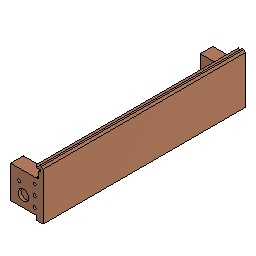
side_right (Autodesk Fusion 360 design; units mm, degrees)
Autodesk Fusion 360 part; units mm, degrees
note: some values were not read from the file. Set by a fixed rule: which sketch regions a step uses.
sketch "Skizze1" plane through (0, 0, 0) normal (0, 1, 0) x (1, 0, 0)
  line L0 (0, -95.7521) -> (0, 79.6341) construction
  line L1 (0, 0) -> (0, -57.828)
  line L2 (-44, 0) -> (25, 0) construction
  line L3 (0, -57.828) -> (-4, -57.828)
  line L4 (-10.2207, -51.6073) -> (4.586, -66.414) construction
  line L5 (-4, -57.828) -> (-6.8284, -54.9996)
  line L6 (-6.8284, -54.9996) -> (-8.243, -56.4141)
  line L7 (-8.243, -56.4141) -> (-8.243, 0)
  line L8 (-8.243, 0) -> (0, 0)
  line L9 (-8.243, -53.585) -> (-5.243, -53.585)
  line L10 (-5.243, -53.585) -> (-3.243, -53.585)
  line L11 (-3.243, -53.585) -> (-3.243, -51.585)
  line L12 (-3.243, -51.585) -> (-5.243, -51.585)
  line L13 (-5.243, -51.585) -> (-5.243, -53.585)
  line L14 (-8.243, -43.585) -> (-12.058, -43.585)
  line L15 (-12.058, -43.585) -> (-8.243, -53.585)
  line L16 (-8.243, -43.585) -> (-5.243, -43.585)
  line L17 (-5.243, -51.585) -> (-5.243, -43.585)
  dimension "d1" = 57.828
  dimension "d2" = 4
  dimension "d3" = 45
  dimension "d4" = 4
  dimension "d5" = 8.243
  dimension "d6" = 4.243
  dimension "d7" = 2
  dimension "d8" = 2
  dimension "d9" = 3
  dimension "d10" = 3.815
  dimension "d11" = 10
  dimension "d17" = 14.243
  dimension "d18" = 43.585
  constraint vertical L0
  constraint coincident L1.start L0
  constraint coincident L1.start L8.end
  constraint coincident L0 L1.end
  constraint horizontal L2
  constraint coincident L1.start L2
  constraint perpendicular L0 L3
  constraint coincident L3.end L4
  constraint coincident L4 L5.end
  constraint perpendicular L5 L6
  constraint vertical L7
  constraint coincident L6.end L7.start
  constraint coincident L2 L7.end
  constraint coincident L7 L9.start
  constraint perpendicular L7 L9
  constraint horizontal L10
  constraint vertical L11
  constraint horizontal L12
  constraint vertical L13
  constraint coincident L7 L14.start
  constraint perpendicular L7 L14
  constraint perpendicular L7 L16
  constraint perpendicular L16 L17
  constraint coincident L16.end L17.end
  measures "d1" distance of L1.end L2
  measures "d2" distance of L0 L3.end
  measures "d3" angle of L0 L4
  measures "d4" distance of L3.end L5.end
  measures "d5" distance of L0 L7
  measures "d6" distance of L3 L9
  measures "d7" distance of L11 L13
  measures "d8" distance of L10 L12
  measures "d9" distance of L7 L9.end
  measures "d10" distance of L7 L14.end
  measures "d11" distance of L9.start L14.start
  measures "d17" distance of L3 L16
  measures "d18" distance of L2 L16.end
extrude "Extrusion1" add sketch "Skizze1" along normal blind 238 contours L1 L3 L5 L6 L7 L8 L9 L10 L11 L12 L16 L17
chamfer "Fase1" distance 2 angle 45 1 edges at (0, 119, 57.828)
ref_plane "Arbeitsebene1" through (-8.243, 0, 0) normal (1, 0, 0) x (0, 1, 0)
sketch "Skizze2" plane through (-8.243, 0, 0) normal (1, 0, 0) x (0, 1, 0)
  line L0 (267.8707, 0) -> (-22.3676, 0) construction
  line L1 (119, 85.1041) -> (119, -43.9964) construction
  line L2 (0, 97.1577) -> (0, -47.4856) construction
  line L3 (274.9535, 43.585) -> (-31.1829, 43.585) construction
  line L4 (115.5, 43.585) -> (122.5, 43.585)
  line L5 (122.5, 43.585) -> (122.5, 50.463)
  line L6 (122.5, 50.463) -> (115.5, 50.463)
  line L7 (115.5, 50.463) -> (115.5, 43.585)
  line L8 (115.5, 43.585) -> (122.5, 50.463) construction
  line L9 (122.5, 43.585) -> (115.5, 50.463) construction
  line L10 (267.9623, 50.463) -> (-13.8401, 50.463) construction
  line L11 (203.5, 43.585) -> (210.5, 43.585)
  line L12 (210.5, 43.585) -> (210.5, 50.463)
  line L13 (210.5, 50.463) -> (203.5, 50.463)
  line L14 (203.5, 50.463) -> (203.5, 43.585)
  line L15 (203.5, 43.585) -> (210.5, 50.463) construction
  line L16 (210.5, 43.585) -> (203.5, 50.463) construction
  line L17 (28.5, 43.585) -> (35.5, 43.585)
  line L18 (35.5, 43.585) -> (35.5, 50.463)
  line L19 (35.5, 50.463) -> (28.5, 50.463)
  line L20 (28.5, 50.463) -> (28.5, 43.585)
  line L21 (28.5, 43.585) -> (35.5, 50.463) construction
  line L22 (35.5, 43.585) -> (28.5, 50.463) construction
  line L23 (220, 68.3899) -> (220, -18.0018) construction
  line L24 (20, 66.908) -> (20, -20) construction
  line L25 (85, 65.5036) -> (85, 11.088) construction
  line L26 (155, 67.0596) -> (155, 11.5194) construction
  line L27 (250.7349, 48.499) -> (-43.738, 48.499) construction
  circle A0 centre (155, 48.499) radius 1.25
  circle A1 centre (85, 48.499) radius 1.25
  circle A2 centre (20, 48.499) radius 1.25
  circle A3 centre (220, 48.499) radius 1.25
  line L28 (21.2702, 46.299) -> (22.5403, 48.499)
  line L29 (22.5403, 48.499) -> (21.2702, 50.699)
  line L30 (21.2702, 50.699) -> (18.7298, 50.699)
  line L31 (18.7298, 50.699) -> (17.4597, 48.499)
  line L32 (17.4597, 48.499) -> (18.7298, 46.299)
  line L33 (18.7298, 46.299) -> (21.2702, 46.299)
  line L34 (86.2702, 46.299) -> (87.5403, 48.499)
  line L35 (87.5403, 48.499) -> (86.2702, 50.699)
  line L36 (86.2702, 50.699) -> (83.7298, 50.699)
  line L37 (83.7298, 50.699) -> (82.4597, 48.499)
  line L38 (82.4597, 48.499) -> (83.7298, 46.299)
  line L39 (83.7298, 46.299) -> (86.2702, 46.299)
  line L40 (156.2702, 46.299) -> (157.5403, 48.499)
  line L41 (157.5403, 48.499) -> (156.2702, 50.699)
  line L42 (156.2702, 50.699) -> (153.7298, 50.699)
  line L43 (153.7298, 50.699) -> (152.4597, 48.499)
  line L44 (152.4597, 48.499) -> (153.7298, 46.299)
  line L45 (153.7298, 46.299) -> (156.2702, 46.299)
  line L46 (221.2702, 46.299) -> (222.5403, 48.499)
  line L47 (222.5403, 48.499) -> (221.2702, 50.699)
  line L48 (221.2702, 50.699) -> (218.7298, 50.699)
  line L49 (218.7298, 50.699) -> (217.4597, 48.499)
  line L50 (217.4597, 48.499) -> (218.7298, 46.299)
  line L51 (218.7298, 46.299) -> (221.2702, 46.299)
  line L52 (238, 80) -> (238, -10) construction
  line L53 (223, 43) -> (223, 20)
  line L54 (223, 20) -> (193, 20)
  line L55 (223, 43) -> (238, 43)
  line L56 (15, 43) -> (0, 43)
  line L57 (15, 43) -> (15, 20)
  line L58 (15, 20) -> (45, 20)
  line L59 (238, 43) -> (238, 5)
  line L60 (238, 5) -> (193, 5)
  line L61 (193, 20) -> (193, 5)
  line L62 (45, 20) -> (45, 5)
  line L63 (0, 5) -> (45, 5)
  line L64 (0, 43) -> (0, 5)
  line L65 (66.5, 43.585) -> (63.5, 43.585) construction
  line L66 (63.5, 43.585) -> (63.5, 48.585)
  line L67 (60.5, 51.585) -> (69.5, 51.585)
  line L68 (66.5, 48.585) -> (66.5, 43.585)
  line L69 (66.5, 43.585) -> (63.5, 43.585) construction
  line L70 (63.5, 43.585) -> (63.5, 33.585)
  line L71 (66.5, 33.585) -> (66.5, 43.585)
  line L72 (65, 56) -> (65, 28) construction
  arc A4 (63.5, 33.585) -> (66.5, 33.585) centre (65, 33.585) ccw
  line L73 (125.8642, 33.585) -> (76, 33.585) construction
  circle A5 centre (58.65, 33.585) radius 4
  circle A6 centre (71.35, 33.585) radius 4
  circle A7 centre (58.65, 33.585) radius 3
  circle A8 centre (71.35, 33.585) radius 3
  line L74 (72.6202, 31.385) -> (73.8903, 33.585)
  line L75 (73.8903, 33.585) -> (72.6202, 35.785)
  line L76 (72.6202, 35.785) -> (70.0798, 35.785)
  line L77 (70.0798, 35.785) -> (68.8097, 33.585)
  line L78 (68.8097, 33.585) -> (70.0798, 31.385)
  line L79 (70.0798, 31.385) -> (72.6202, 31.385)
  line L80 (59.9202, 31.385) -> (61.1903, 33.585)
  line L81 (61.1903, 33.585) -> (59.9202, 35.785)
  line L82 (59.9202, 35.785) -> (57.3798, 35.785)
  line L83 (57.3798, 35.785) -> (56.1097, 33.585)
  line L84 (56.1097, 33.585) -> (57.3798, 31.385)
  line L85 (57.3798, 31.385) -> (59.9202, 31.385)
  circle A9 centre (71.35, 33.585) radius 1.25
  circle A10 centre (58.65, 33.585) radius 1.25
  arc A11 (69.5, 51.585) -> (66.5, 48.585) centre (69.5, 48.585) ccw
  arc A12 (63.5, 48.585) -> (60.5, 51.585) centre (60.5, 48.585) ccw
  line L86 (192, 26.585) -> (129, 26.585) construction
  line L87 (99, 16.585) -> (129, 16.585) construction
  line L88 (129, 16.585) -> (129, 36.585) construction
  line L89 (129, 36.585) -> (99, 36.585) construction
  line L90 (99, 36.585) -> (99, 16.585) construction
  line L91 (129, 36.585) -> (139, 36.585) construction
  line L92 (139, 36.585) -> (139, 16.585) construction
  line L93 (139, 16.585) -> (129, 16.585) construction
  line L94 (129, 16.585) -> (129, 36.585) construction
  circle A13 centre (99, 26.585) radius 1.25
  circle A14 centre (99, 26.585) radius 4
  circle A15 centre (129, 16.585) radius 1.25
  circle A16 centre (129, 16.585) radius 4
  circle A17 centre (129, 36.585) radius 1.25
  circle A18 centre (129, 36.585) radius 4
  line L95 (130.2702, 34.385) -> (131.5403, 36.585)
  line L96 (131.5403, 36.585) -> (130.2702, 38.785)
  line L97 (130.2702, 38.785) -> (127.7298, 38.785)
  line L98 (127.7298, 38.785) -> (126.4597, 36.585)
  line L99 (126.4597, 36.585) -> (127.7298, 34.385)
  line L100 (127.7298, 34.385) -> (130.2702, 34.385)
  line L101 (130.2702, 14.385) -> (131.5403, 16.585)
  line L102 (131.5403, 16.585) -> (130.2702, 18.785)
  line L103 (130.2702, 18.785) -> (127.7298, 18.785)
  line L104 (127.7298, 18.785) -> (126.4597, 16.585)
  line L105 (126.4597, 16.585) -> (127.7298, 14.385)
  line L106 (127.7298, 14.385) -> (130.2702, 14.385)
  line L107 (100.2702, 24.385) -> (101.5403, 26.585)
  line L108 (101.5403, 26.585) -> (100.2702, 28.785)
  line L109 (100.2702, 28.785) -> (97.7298, 28.785)
  line L110 (97.7298, 28.785) -> (96.4597, 26.585)
  line L111 (96.4597, 26.585) -> (97.7298, 24.385)
  line L112 (97.7298, 24.385) -> (100.2702, 24.385)
  line L113 (99, 36.585) -> (129, 16.585) construction
  line L114 (129, 36.585) -> (99, 16.585) construction
  point P0 (119, 47.024)
  point P1 (207, 47.024)
  point P2 (32, 47.024)
  point P3 (20, 48.499)
  point P4 (85, 48.499)
  point P5 (155, 48.499)
  point P6 (220, 48.499)
  point P7 (68.35, 33.585)
  point P8 (61.65, 33.585)
  point P9 (71.35, 33.585)
  point P10 (58.65, 33.585)
  point P11 (155, 26.585)
  point P12 (129, 36.585)
  point P13 (129, 16.585)
  point P14 (99, 26.585)
  point P15 (114, 26.585)
  dimension "d16" = 119
  dimension "d19" = 43.585
  dimension "d20" = 7
  dimension "d22" = 6.878
  dimension "d23" = 7
  dimension "d24" = 7
  dimension "d25" = 88
  dimension "d26" = 87
  dimension "d27" = 101
  dimension "d28" = 99
  dimension "d30" = 34
  dimension "d32" = 36
  dimension "d33" = 4.914
  dimension "d34" = 2.5
  dimension "d35" = 2.5
  dimension "d36" = 2.5
  dimension "d37" = 2.5
  dimension "d38" = 4.4
  dimension "d39" = 4.4
  dimension "d40" = 4.4
  dimension "d41" = 4.4
  dimension "d42" = 119
  dimension "d60" = 15
  dimension "d61" = 38
  dimension "d62" = 5
  dimension "d63" = 15
  dimension "d64" = 45
  dimension "d154" = 8
  dimension "d155" = 3
  dimension "d157" = 1.5
  dimension "d159" = 1.5
  dimension "d162" = 6.35
  dimension "d163" = 8
  dimension "d164" = 10
  dimension "d165" = 6.35
  dimension "d166" = 8
  dimension "d167" = 6
  dimension "d168" = 6
  dimension "d169" = 4.4
  dimension "d170" = 4.4
  dimension "d171" = 2.5
  dimension "d172" = 2.5
  dimension "d177" = 3
  dimension "d178" = 3
  dimension "d189" = 20
  dimension "d190" = 30
  dimension "d191" = 10
  dimension "d192" = 17
  dimension "d193" = 8
  dimension "d194" = 8
  dimension "d195" = 8
  dimension "d196" = 2.5
  dimension "d197" = 2.5
  dimension "d198" = 2.5
  dimension "d199" = 4.4
  dimension "d200" = 4.4
  dimension "d201" = 4.4
  dimension "d204" = 20
  dimension "d205" = 5
  constraint horizontal L0
  constraint coincident origin L0
  constraint perpendicular L0 L1
  constraint perpendicular L0 L2
  constraint coincident origin L2
  constraint perpendicular L1 L3
  constraint horizontal L4
  constraint perpendicular L4 L5
  constraint parallel L4 L6
  constraint parallel L5 L7
  constraint coincident L8 P0
  constraint coincident L9 P0
  constraint coincident L1 P0
  constraint coincident L3 L4.start
  constraint perpendicular L2 L10
  constraint coincident L6.end L10
  constraint horizontal L11
  constraint perpendicular L11 L12
  constraint parallel L11 L13
  constraint parallel L12 L14
  constraint coincident L15 P1
  constraint coincident L16 P1
  constraint horizontal L17
  constraint perpendicular L17 L18
  constraint parallel L17 L19
  constraint parallel L18 L20
  constraint coincident L21 P2
  constraint coincident L22 P2
  constraint coincident L3 L17.start
  constraint coincident L10 L18.end
  constraint coincident L3 L11.start
  constraint coincident L10 L13.end
  constraint perpendicular L3 L23
  constraint perpendicular L10 L24
  constraint perpendicular L10 L25
  constraint perpendicular L3 L26
  constraint perpendicular L2 L27
  constraint coincident L27 P5
  constraint coincident L26 P5
  constraint coincident L27 P4
  constraint coincident L25 P4
  constraint coincident L24 P3
  constraint coincident L27 P3
  constraint coincident L27 P6
  constraint coincident L23 P6
  constraint coincident P3 A2.centre
  constraint coincident P4 A1.centre
  constraint coincident P5 A0.centre
  constraint coincident P6 A3.centre
  constraint horizontal L51
  constraint horizontal L45
  constraint horizontal L39
  constraint horizontal L33
  constraint perpendicular L27 L52
  constraint coincident L52 L55.end
  constraint perpendicular L0 L53
  constraint perpendicular L53 L54
  constraint symmetric L1 L55.end L56.end
  constraint symmetric L1 L53.start L56.start
  constraint symmetric L1 L53.end L57.end
  constraint symmetric L1 L54.end L58.end
  constraint coincident L52 L59.end
  constraint perpendicular L55 L59
  constraint perpendicular L59 L60
  constraint perpendicular L60 L61
  constraint coincident L60.end L61.end
  constraint symmetric L1 L59.end L63.start
  constraint symmetric L1 L60.end L62.end
  constraint horizontal L65
  constraint vertical L66
  constraint horizontal L67
  constraint vertical L68
  constraint coincident L3 L65.start
  constraint horizontal L69
  constraint vertical L70
  constraint vertical L71
  constraint coincident L66 L65.end
  constraint perpendicular L25 L73
  constraint coincident A4.centre L73
  constraint coincident L73 P10
  constraint coincident L71.start L73
  constraint coincident L73 P9
  constraint concentric A5 A7
  constraint concentric A6 A8
  constraint coincident L73 P7
  constraint coincident A8 P7
  constraint coincident L73 P8
  constraint coincident A7 P8
  constraint coincident P9 A6.centre
  constraint coincident P10 A5.centre
  constraint horizontal L85
  constraint horizontal L79
  constraint concentric A8 A9
  constraint concentric A5 A10
  constraint tangent L67 A12
  constraint tangent L66 A12
  constraint tangent L68 A11
  constraint tangent L67 A11
  constraint perpendicular L26 L86
  constraint horizontal L87
  constraint perpendicular L87 L88
  constraint parallel L87 L89
  constraint parallel L88 L90
  constraint coincident L86 P11
  constraint horizontal L91
  constraint vertical L92
  constraint horizontal L93
  constraint vertical L94
  constraint coincident L87 P13
  constraint coincident L26 P11
  constraint midpoint L90 P14
  constraint concentric A13 A14
  constraint coincident P13 L87.end
  constraint concentric A15 A16
  constraint coincident P12 L88.end
  constraint concentric A17 A18
  constraint coincident P14 A13.centre
  constraint horizontal L112
  constraint horizontal L100
  constraint horizontal L106
  constraint midpoint L114 P15
  constraint coincident L86 P15
  measures "d16" distance of L1 L2
  measures "d19" distance of L0 L3
  measures "d20" distance of L5 L7
  measures "d22" distance of L3 L10
  measures "d23" distance of L18 L20
  measures "d24" distance of L12 L14
  measures "d25" distance of L1 P1
  measures "d26" distance of L1 P2
  measures "d27" distance of L1 L23
  measures "d28" distance of L1 L24
  measures "d30" distance of L1 L25
  measures "d32" distance of L1 L26
  measures "d33" distance of L3 L27
  measures "d34" diameter of A3
  measures "d35" diameter of A0
  measures "d36" diameter of A1
  measures "d37" diameter of A2
  measures "d38" distance of L30 L33
  measures "d39" distance of L36 L39
  measures "d40" distance of L42 L45
  measures "d41" distance of L48 L51
  measures "d42" distance of L1 L52
  measures "d60" distance of L54 L60
  measures "d61" distance of L55 L60
  measures "d62" distance of L0 L60
  measures "d63" distance of L53 L59
  measures "d64" distance of L52 L61
  measures "d154" distance of L65 L67
  measures "d155" distance of L66 L68
  measures "d157" distance of L71 L72
  measures "d159" radius of A4
  measures "d162" distance of A4.centre P10
  measures "d163" diameter of A5
  measures "d164" distance of L3 L73
  measures "d165" distance of L72 P9
  measures "d166" diameter of A6
  measures "d167" diameter of A7
  measures "d168" diameter of A8
  measures "d169" distance of L76 L79
  measures "d170" distance of L82 L85
  measures "d171" diameter of A10
  measures "d172" diameter of A9
  measures "d177" radius of A12
  measures "d178" radius of A11
  measures "d189" distance of L87 L89
  measures "d190" distance of L88 L90
  measures "d191" distance of L88 L92
  measures "d192" distance of L3 L86
  measures "d193" diameter of A14
  measures "d194" diameter of A16
  measures "d195" diameter of A18
  measures "d196" diameter of A17
  measures "d197" diameter of A15
  measures "d198" diameter of A13
  measures "d199" distance of L109 L112
  measures "d200" distance of L97 L100
  measures "d201" distance of L103 L106
  measures "d204" distance of L25 L72
  measures "d205" distance of L1 P15
extrude "Extrusion2" cut sketch "Skizze2" along normal blind 5 contours L4 L5 L6 L7 | L11 L12 L13 L14 | L17 L18 L19 L20
move_face "Flächen versetzen1" offset -0.2 13 faces at (-7.243, 149.5, 43.585) (-3.243, 33.1667, 45.8777) (-3.243, 117.8333, 48.1703) (-3.243, 208.1667, 48.1703) (-4.5763, 28.5, 48.1703) (-4.5763, 115.5, 48.1703) (-4.5763, 203.5, 48.1703) (-3.9097, 35.5, 48.1703) (-3.9097, 122.5, 48.1703) (-4.5763, 210.5, 48.1703) (-4.5763, 208.1667, 50.463) (-4.5763, 120.1667, 50.463) (-4.5763, 33.1667, 50.463)
extrude "Extrusion3" cut sketch "Skizze2" along normal blind 7 contours A0 | A1 | A2 | A3
extrude "Extrusion4" cut sketch "Skizze2" along normal blind 7 contours L28 L29 L30 L31 L32 L33 | L34 L35 L36 L37 L38 L39 | L40 L41 L42 L43 L44 L45 | L46 L47 L48 L49 L50 L51
extrude "Extrusion5" add sketch "Skizze2" along normal blind 5.2 contours L28 L29 L30 L31 L32 L33 | L34 L35 L36 L37 L38 L39 | L40 L41 L42 L43 L44 L45 | L46 L47 L48 L49 L50 L51
extrude "Extrusion6" cut sketch "Skizze2" along normal blind 3 contours L28 L29 L30 L31 L32 L33 | L34 L35 L36 L37 L38 L39 | L40 L41 L42 L43 L44 L45 | L46 L47 L48 L49 L50 L51
extrude "Extrusion7" add sketch "Skizze2" against normal blind 30 contours L53 L54 L55 L59 L60 L61 | L56 L57 L58 L62 L63 L64
sketch "Skizze3" plane through (0, 0, 0) normal (0, 1, 0) x (1, 0, 0)
  line L0 (0, -92.2199) -> (0, 12.1785) construction
  line L1 (-68.4756, 0) -> (32.4309, 0) construction
  line L2 (-10, -63.9149) -> (-10, 13.2124) construction
  line L3 (-23, -32.8986) -> (-23, 10) construction
  line L4 (-28.243, -73.6203) -> (-28.243, -17.2743) construction
  circle A0 centre (-10, -12) radius 1.75
  circle A1 centre (-10, -24) radius 1.75
  circle A2 centre (-10, -36) radius 1.75
  line L5 (-11.6743, -33.1) -> (-13.3486, -36)
  line L6 (-13.3486, -36) -> (-11.6743, -38.9)
  line L7 (-11.6743, -38.9) -> (-8.3257, -38.9)
  line L8 (-8.3257, -38.9) -> (-6.6514, -36)
  line L9 (-6.6514, -36) -> (-8.3257, -33.1)
  line L10 (-8.3257, -33.1) -> (-11.6743, -33.1)
  line L11 (-11.6743, -21.1) -> (-13.3486, -24)
  line L12 (-13.3486, -24) -> (-11.6743, -26.9)
  line L13 (-11.6743, -26.9) -> (-8.3257, -26.9)
  line L14 (-8.3257, -26.9) -> (-6.6514, -24)
  line L15 (-6.6514, -24) -> (-8.3257, -21.1)
  line L16 (-8.3257, -21.1) -> (-11.6743, -21.1)
  line L17 (-11.6743, -9.1) -> (-13.3486, -12)
  line L18 (-13.3486, -12) -> (-11.6743, -14.9)
  line L19 (-11.6743, -14.9) -> (-8.3257, -14.9)
  line L20 (-8.3257, -14.9) -> (-6.6514, -12)
  line L21 (-6.6514, -12) -> (-8.3257, -9.1)
  line L22 (-8.3257, -9.1) -> (-11.6743, -9.1)
  circle A3 centre (-23, -18) radius 6
  circle A4 centre (-28.243, -30) radius 1.75
  line L23 (-29.9173, -27.1) -> (-31.5916, -30)
  line L24 (-31.5916, -30) -> (-29.9173, -32.9)
  line L25 (-29.9173, -32.9) -> (-26.5687, -32.9)
  line L26 (-26.5687, -32.9) -> (-24.8944, -30)
  line L27 (-24.8944, -30) -> (-26.5687, -27.1)
  line L28 (-26.5687, -27.1) -> (-29.9173, -27.1)
  line L29 (-11.6743, -38.9) -> (-13.3486, -38.9)
  line L30 (-13.3486, -38.9) -> (-13.3486, -33.1)
  line L31 (-13.3486, -33.1) -> (-11.6743, -33.1)
  line L32 (-11.6743, -26.9) -> (-13.3486, -26.9)
  line L33 (-13.3486, -26.9) -> (-13.3486, -21.1)
  line L34 (-13.3486, -21.1) -> (-11.6743, -21.1)
  line L35 (-11.6743, -14.9) -> (-13.3486, -14.9)
  line L36 (-13.3486, -14.9) -> (-13.3486, -9.1)
  line L37 (-13.3486, -9.1) -> (-11.6743, -9.1)
  line L38 (-29.9173, -32.9) -> (-31.5916, -32.9)
  line L39 (-31.5916, -32.9) -> (-31.5916, -27.1)
  line L40 (-31.5916, -27.1) -> (-29.9173, -27.1)
  point P0 (-10, -36)
  point P1 (-10, -24)
  point P2 (-10, -12)
  point P3 (-23, -18)
  point P4 (-28.243, -30)
  dimension "d65" = 10
  dimension "d66" = 13
  dimension "d67" = 28.243
  dimension "d68" = 12
  dimension "d69" = 12
  dimension "d70" = 12
  dimension "d71" = 3.5
  dimension "d72" = 3.5
  dimension "d73" = 3.5
  dimension "d74" = 5.8
  dimension "d75" = 5.8
  dimension "d76" = 5.8
  dimension "d78" = 12
  dimension "d79" = 18
  dimension "d81" = 3.5
  dimension "d82" = 30
  dimension "d83" = 5.8
  constraint vertical L0
  constraint horizontal L1
  constraint coincident origin L0
  constraint coincident origin L1
  constraint perpendicular L1 L2
  constraint perpendicular L1 L3
  constraint vertical L4
  constraint coincident L2 P2
  constraint coincident L2 P1
  constraint coincident L2 P0
  constraint coincident P0 A2.centre
  constraint coincident P1 A1.centre
  constraint coincident P2 A0.centre
  constraint horizontal L10
  constraint horizontal L16
  constraint horizontal L22
  constraint coincident P3 A3.centre
  constraint coincident L4 P4
  constraint coincident P4 A4.centre
  constraint horizontal L28
  constraint horizontal L29
  constraint vertical L30
  constraint horizontal L31
  constraint horizontal L32
  constraint vertical L33
  constraint horizontal L34
  constraint horizontal L35
  constraint vertical L36
  constraint horizontal L37
  constraint horizontal L38
  constraint vertical L39
  constraint horizontal L40
  constraint coincident L28 L23.start
  constraint coincident L10 L5.start
  constraint coincident L16 L11.start
  constraint coincident L22 L17.start
  constraint coincident L17.end L36
  constraint coincident L11.end L33
  constraint coincident L5.end L30
  constraint coincident L23.end L39
  measures "d65" distance of L0 L2
  measures "d66" distance of L2 L3
  measures "d67" distance of L0 L4
  measures "d68" distance of L1 P2
  measures "d69" distance of P2 P1
  measures "d70" distance of P1 P0
  measures "d71" diameter of A2
  measures "d72" diameter of A1
  measures "d73" diameter of A0
  measures "d74" distance of L19 L22
  measures "d75" distance of L13 L16
  measures "d76" distance of L7 L10
  measures "d78" diameter of A3
  measures "d79" distance of L1 P3
  measures "d81" diameter of A4
  measures "d82" distance of L1 P4
  measures "d83" distance of L25 L28
ref_plane "Arbeitsebene2" through (0, 238, 0) normal (0, 1, 0) x (0, 0, 1)
sketch "Skizze4" plane through (0, 238, 0) normal (0, 1, 0) x (1, 0, 0)
  line L0 (0, -55.469) -> (0, 11.8199) construction
  line L1 (5.4144, 0) -> (-61.5509, 0) construction
  line L2 (-10, -43.3376) -> (-10, 10) construction
  circle A0 centre (-10, -12) radius 1.75
  circle A1 centre (-10, -24) radius 1.75
  circle A2 centre (-10, -36) radius 1.75
  line L3 (-28.243, -50) -> (-28.243, 7) construction
  line L4 (-23, -24.4157) -> (-23, -9.4157) construction
  circle A3 centre (-23, -18) radius 6
  circle A4 centre (-28.243, -30) radius 1.75
  line L5 (-11.6743, -33.1) -> (-13.3486, -36)
  line L6 (-13.3486, -36) -> (-11.6743, -38.9)
  line L7 (-11.6743, -38.9) -> (-8.3257, -38.9)
  line L8 (-8.3257, -38.9) -> (-6.6514, -36)
  line L9 (-6.6514, -36) -> (-8.3257, -33.1)
  line L10 (-8.3257, -33.1) -> (-11.6743, -33.1)
  line L11 (-11.6743, -21.1) -> (-13.3486, -24)
  line L12 (-13.3486, -24) -> (-11.6743, -26.9)
  line L13 (-11.6743, -26.9) -> (-8.3257, -26.9)
  line L14 (-8.3257, -26.9) -> (-6.6514, -24)
  line L15 (-6.6514, -24) -> (-8.3257, -21.1)
  line L16 (-8.3257, -21.1) -> (-11.6743, -21.1)
  line L17 (-11.6743, -9.1) -> (-13.3486, -12)
  line L18 (-13.3486, -12) -> (-11.6743, -14.9)
  line L19 (-11.6743, -14.9) -> (-8.3257, -14.9)
  line L20 (-8.3257, -14.9) -> (-6.6514, -12)
  line L21 (-6.6514, -12) -> (-8.3257, -9.1)
  line L22 (-8.3257, -9.1) -> (-11.6743, -9.1)
  line L23 (-29.9173, -27.1) -> (-31.5916, -30)
  line L24 (-31.5916, -30) -> (-29.9173, -32.9)
  line L25 (-29.9173, -32.9) -> (-26.5687, -32.9)
  line L26 (-26.5687, -32.9) -> (-24.8944, -30)
  line L27 (-24.8944, -30) -> (-26.5687, -27.1)
  line L28 (-26.5687, -27.1) -> (-29.9173, -27.1)
  line L29 (-11.6743, -38.9) -> (-13.3486, -38.9)
  line L30 (-13.3486, -38.9) -> (-13.3486, -33.1)
  line L31 (-13.3486, -33.1) -> (-11.6743, -33.1)
  line L32 (-11.6743, -33.1) -> (-11.6743, -38.9)
  line L33 (-11.6743, -26.9) -> (-13.3486, -26.9)
  line L34 (-13.3486, -26.9) -> (-13.3486, -21.1)
  line L35 (-13.3486, -21.1) -> (-11.6743, -21.1)
  line L36 (-11.6743, -21.1) -> (-11.6743, -26.9)
  line L37 (-11.6743, -14.9) -> (-13.3486, -14.9)
  line L38 (-13.3486, -14.9) -> (-13.3486, -9.1)
  line L39 (-13.3486, -9.1) -> (-11.6743, -9.1)
  line L40 (-11.6743, -9.1) -> (-11.6743, -14.9)
  line L41 (-29.9173, -32.9) -> (-31.5916, -32.9)
  line L42 (-31.5916, -32.9) -> (-31.5916, -27.1)
  line L43 (-31.5916, -27.1) -> (-29.9173, -27.1)
  line L44 (-29.9173, -27.1) -> (-29.9173, -32.9)
  point P0 (-10, -36)
  point P1 (-10, -24)
  point P2 (-10, -12)
  point P3 (-28.243, -30)
  dimension "d94" = 10
  dimension "d95" = 12
  dimension "d96" = 12
  dimension "d97" = 12
  dimension "d98" = 3.5
  dimension "d99" = 3.5
  dimension "d100" = 3.5
  dimension "d101" = 28.243
  dimension "d102" = 13
  dimension "d103" = 12
  dimension "d104" = 18
  dimension "d105" = 3.5
  dimension "d106" = 30
  dimension "d107" = 5.8
  dimension "d108" = 5.8
  dimension "d109" = 5.8
  dimension "d110" = 5.8
  constraint vertical L0
  constraint coincident origin L0
  constraint horizontal L1
  constraint coincident origin L1
  constraint perpendicular L1 L2
  constraint coincident L2 P2
  constraint coincident L2 P1
  constraint coincident L2 P0
  constraint perpendicular L1 L3
  constraint vertical L4
  constraint coincident L4 A3.centre
  constraint coincident L3 P3
  constraint coincident P0 A2.centre
  constraint coincident P1 A1.centre
  constraint coincident P2 A0.centre
  constraint coincident P3 A4.centre
  constraint horizontal L10
  constraint horizontal L16
  constraint horizontal L22
  constraint horizontal L28
  constraint horizontal L29
  constraint vertical L30
  constraint horizontal L31
  constraint vertical L32
  constraint horizontal L33
  constraint vertical L34
  constraint horizontal L35
  constraint vertical L36
  constraint horizontal L37
  constraint vertical L38
  constraint horizontal L39
  constraint vertical L40
  constraint horizontal L41
  constraint vertical L42
  constraint horizontal L43
  constraint vertical L44
  constraint coincident L28 L23.start
  constraint coincident L23.end L42
  constraint coincident L5.end L30
  constraint coincident L10 L5.start
  constraint coincident L16 L11.start
  constraint coincident L11.end L34
  constraint coincident L17.end L38
  constraint coincident L22 L17.start
  measures "d94" distance of L0 L2
  measures "d95" distance of L1 P2
  measures "d96" distance of P2 P1
  measures "d97" distance of P1 P0
  measures "d98" diameter of A0
  measures "d99" diameter of A1
  measures "d100" diameter of A2
  measures "d101" distance of L0 L3
  measures "d102" distance of L2 L4
  measures "d103" diameter of A3
  measures "d104" distance of L1 A3.centre
  measures "d105" diameter of A4
  measures "d106" distance of L1 P3
  measures "d107" distance of L25 L28
  measures "d108" distance of L19 L22
  measures "d109" distance of L13 L16
  measures "d110" distance of L7 L10
extrude "Extrusion8" cut sketch "Skizze3" along normal blind 3 contours A3
extrude "Extrusion12" cut sketch "Skizze4" against normal blind 3 contours A3
move_face "Flächen versetzen2" offset -0.2 2 faces at (-21.235, 3, 16.6397) (-17.0075, 2, 18.2991)
move_face "Flächen versetzen3" offset -0.2 2 faces at (-21.235, 235, 16.6397) (-17.0075, 236, 18.2991)
extrude "Extrusion9" cut sketch "Skizze3" along normal blind 17 contours A0 | A1 | A2 | A4
extrude "Extrusion13" cut sketch "Skizze4" against normal blind 17 contours A0 L40 | A0 L40 | A1 L36 | A1 L36 | A2 L32 | A2 L32 | A4 L44 | A4 L44
extrude "Extrusion10" cut sketch "Skizze3" along normal blind 6 contours L5 L6 L7 L8 L9 L10 | L5 L30 L31 | L6 L29 L30 | L11 L12 L13 L14 L15 L16 | L11 L33 L34 | L12 L32 L33 | L17 L18 L19 L20 L21 L22 | L17 L36 L37 | L18 L35 L36 | L23 L24 L25 L26 L27 L28 | L23 L39 L40 | L24 L38 L39
extrude "Extrusion14" cut sketch "Skizze4" against normal blind 6 contours A0 L19 L20 L21 L22 L40 | A0 L17 L18 L40 | L17 L38 L39 | L18 L37 L38 | A1 L13 L14 L15 L16 L36 | A1 L11 L12 L36 | L11 L34 L35 | L12 L33 L34 | A2 L7 L8 L9 L10 L32 | A2 L5 L6 L32 | L5 L30 L31 | L6 L29 L30 | A4 L25 L26 L27 L28 L44 | A4 L23 L24 L44 | L23 L42 L43 | L24 L41 L42
extrude "Extrusion11" add sketch "Skizze3" along normal blind 3.2 contours L5 L6 L7 L8 L9 L10 | L5 L30 L31 | L6 L29 L30 | L11 L12 L13 L14 L15 L16 | L11 L33 L34 | L12 L32 L33 | L17 L18 L19 L20 L21 L22 | L17 L36 L37 | L18 L35 L36 | L23 L24 L25 L26 L27 L28 | L23 L39 L40 | L24 L38 L39
extrude "Extrusion15" add sketch "Skizze4" against normal blind 3.2 contours A0 L19 L20 L21 L22 L40 | A0 L17 L18 L40 | L17 L38 L39 | L18 L37 L38 | A1 L13 L14 L15 L16 L36 | A1 L11 L12 L36 | L11 L34 L35 | L12 L33 L34 | A2 L7 L8 L9 L10 L32 | A2 L5 L6 L32 | L5 L30 L31 | L6 L29 L30 | A4 L25 L26 L27 L28 L44 | A4 L23 L24 L44 | L23 L42 L43 | L24 L41 L42
ref_plane "Arbeitsebene3" through (0, 0, 5) normal (0, 0, 1) x (1, 0, 0)
sketch "Skizze5" plane through (0, 0, 5) normal (0, 0, 1) x (1, 0, 0)
  line L0 (0, 304.2295) -> (0, -44.6132) construction
  line L1 (40.8968, 0) -> (-125, 0) construction
  line L2 (-16.743, 290) -> (-16.743, -30) construction
  line L3 (-30.743, 288.1348) -> (-30.743, -30) construction
  line L4 (17.6636, 10) -> (-56.9116, 10) construction
  line L5 (15.9426, 35) -> (-60, 35) construction
  line L6 (28.5025, 203) -> (-55.3761, 203) construction
  line L7 (20, 228) -> (-65.678, 228) construction
  line L8 (-12.2276, 194.9367) -> (-36.234, 237.8054) construction
  line L9 (-7.0433, 245.3209) -> (-37.9735, 190.0885) construction
  line L10 (-12.4101, 42.7373) -> (-35.0759, 2.2627) construction
  line L11 (-13.8411, 4.818) -> (-37.2196, 46.5654) construction
  circle A0 centre (-23.743, 22.5) radius 4
  circle A1 centre (-23.743, 215.5) radius 4
  circle A2 centre (-30.743, 10) radius 1.75
  circle A3 centre (-30.743, 35) radius 1.75
  circle A4 centre (-16.743, 35) radius 1.75
  circle A5 centre (-16.743, 10) radius 1.75
  circle A6 centre (-30.743, 228) radius 1.75
  circle A7 centre (-16.743, 228) radius 1.75
  circle A8 centre (-16.743, 203) radius 1.75
  circle A9 centre (-30.743, 203) radius 1.75
  line L12 (-29.0687, 225.1) -> (-27.3944, 228)
  line L13 (-27.3944, 228) -> (-29.0687, 230.9)
  line L14 (-29.0687, 230.9) -> (-32.4173, 230.9)
  line L15 (-32.4173, 230.9) -> (-34.0916, 228)
  line L16 (-34.0916, 228) -> (-32.4173, 225.1)
  line L17 (-32.4173, 225.1) -> (-29.0687, 225.1)
  line L18 (-15.0687, 225.1) -> (-13.3944, 228)
  line L19 (-13.3944, 228) -> (-15.0687, 230.9)
  line L20 (-15.0687, 230.9) -> (-18.4173, 230.9)
  line L21 (-18.4173, 230.9) -> (-20.0916, 228)
  line L22 (-20.0916, 228) -> (-18.4173, 225.1)
  line L23 (-18.4173, 225.1) -> (-15.0687, 225.1)
  line L24 (-15.0687, 200.1) -> (-13.3944, 203)
  line L25 (-13.3944, 203) -> (-15.0687, 205.9)
  line L26 (-15.0687, 205.9) -> (-18.4173, 205.9)
  line L27 (-18.4173, 205.9) -> (-20.0916, 203)
  line L28 (-20.0916, 203) -> (-18.4173, 200.1)
  line L29 (-18.4173, 200.1) -> (-15.0687, 200.1)
  line L30 (-29.0687, 200.1) -> (-27.3944, 203)
  line L31 (-27.3944, 203) -> (-29.0687, 205.9)
  line L32 (-29.0687, 205.9) -> (-32.4173, 205.9)
  line L33 (-32.4173, 205.9) -> (-34.0916, 203)
  line L34 (-34.0916, 203) -> (-32.4173, 200.1)
  line L35 (-32.4173, 200.1) -> (-29.0687, 200.1)
  line L36 (-29.0687, 32.1) -> (-27.3944, 35)
  line L37 (-27.3944, 35) -> (-29.0687, 37.9)
  line L38 (-29.0687, 37.9) -> (-32.4173, 37.9)
  line L39 (-32.4173, 37.9) -> (-34.0916, 35)
  line L40 (-34.0916, 35) -> (-32.4173, 32.1)
  line L41 (-32.4173, 32.1) -> (-29.0687, 32.1)
  line L42 (-15.0687, 32.1) -> (-13.3944, 35)
  line L43 (-13.3944, 35) -> (-15.0687, 37.9)
  line L44 (-15.0687, 37.9) -> (-18.4173, 37.9)
  line L45 (-18.4173, 37.9) -> (-20.0916, 35)
  line L46 (-20.0916, 35) -> (-18.4173, 32.1)
  line L47 (-18.4173, 32.1) -> (-15.0687, 32.1)
  line L48 (-15.0687, 7.1) -> (-13.3944, 10)
  line L49 (-13.3944, 10) -> (-15.0687, 12.9)
  line L50 (-15.0687, 12.9) -> (-18.4173, 12.9)
  line L51 (-18.4173, 12.9) -> (-20.0916, 10)
  line L52 (-20.0916, 10) -> (-18.4173, 7.1)
  line L53 (-18.4173, 7.1) -> (-15.0687, 7.1)
  line L54 (-29.0687, 7.1) -> (-27.3944, 10)
  line L55 (-27.3944, 10) -> (-29.0687, 12.9)
  line L56 (-29.0687, 12.9) -> (-32.4173, 12.9)
  line L57 (-32.4173, 12.9) -> (-34.0916, 10)
  line L58 (-34.0916, 10) -> (-32.4173, 7.1)
  line L59 (-32.4173, 7.1) -> (-29.0687, 7.1)
  line L60 (-18.4173, 12.9) -> (-20.0916, 12.9)
  line L61 (-20.0916, 12.9) -> (-20.0916, 7.1)
  line L62 (-20.0916, 7.1) -> (-18.4173, 7.1)
  line L63 (-18.4173, 7.1) -> (-18.4173, 12.9)
  line L64 (-32.4173, 12.9) -> (-34.0916, 12.9)
  line L65 (-34.0916, 12.9) -> (-34.0916, 7.1)
  line L66 (-34.0916, 7.1) -> (-32.4173, 7.1)
  line L67 (-32.4173, 7.1) -> (-32.4173, 12.9)
  line L68 (-32.4173, 37.9) -> (-34.0916, 37.9)
  line L69 (-34.0916, 37.9) -> (-34.0916, 32.1)
  line L70 (-34.0916, 32.1) -> (-32.4173, 32.1)
  line L71 (-32.4173, 32.1) -> (-32.4173, 37.9)
  line L72 (-18.4173, 37.9) -> (-20.0916, 37.9)
  line L73 (-20.0916, 37.9) -> (-20.0916, 32.1)
  line L74 (-20.0916, 32.1) -> (-18.4173, 32.1)
  line L75 (-18.4173, 32.1) -> (-18.4173, 37.9)
  line L76 (-18.4173, 205.9) -> (-20.0916, 205.9)
  line L77 (-20.0916, 205.9) -> (-20.0916, 200.1)
  line L78 (-20.0916, 200.1) -> (-18.4173, 200.1)
  line L79 (-18.4173, 200.1) -> (-18.4173, 205.9)
  line L80 (-32.4173, 205.9) -> (-34.0916, 205.9)
  line L81 (-34.0916, 205.9) -> (-34.0916, 200.1)
  line L82 (-34.0916, 200.1) -> (-32.4173, 200.1)
  line L83 (-32.4173, 200.1) -> (-32.4173, 205.9)
  line L84 (-32.4173, 230.9) -> (-34.0916, 230.9)
  line L85 (-34.0916, 230.9) -> (-34.0916, 225.1)
  line L86 (-34.0916, 225.1) -> (-32.4173, 225.1)
  line L87 (-32.4173, 225.1) -> (-32.4173, 230.9)
  line L88 (-18.4173, 230.9) -> (-20.0916, 230.9)
  line L89 (-20.0916, 230.9) -> (-20.0916, 225.1)
  line L90 (-20.0916, 225.1) -> (-18.4173, 225.1)
  line L91 (-18.4173, 225.1) -> (-18.4173, 230.9)
  point P0 (-16.743, 203)
  point P1 (-16.743, 228)
  point P2 (-23.743, 215.5)
  point P3 (-30.743, 228)
  point P4 (-30.743, 203)
  point P5 (-16.743, 35)
  point P6 (-30.743, 35)
  point P7 (-30.743, 10)
  point P8 (-16.743, 10)
  point P9 (-23.743, 22.5)
  point P10 (-30.743, 228)
  point P11 (-16.743, 228)
  point P12 (-16.743, 203)
  point P13 (-30.743, 203)
  point P14 (-30.743, 35)
  point P15 (-16.743, 35)
  point P16 (-16.743, 10)
  point P17 (-30.743, 10)
  dimension "d121" = 16.743
  dimension "d122" = 14
  dimension "d123" = 10
  dimension "d124" = 25
  dimension "d125" = 168
  dimension "d126" = 25
  dimension "d127" = 8
  dimension "d128" = 8
  dimension "d129" = 3.5
  dimension "d130" = 3.5
  dimension "d131" = 3.5
  dimension "d132" = 3.5
  dimension "d133" = 3.5
  dimension "d134" = 3.5
  dimension "d135" = 3.5
  dimension "d136" = 3.5
  dimension "d137" = 5.8
  dimension "d138" = 5.8
  dimension "d139" = 5.8
  dimension "d140" = 5.8
  dimension "d141" = 5.8
  dimension "d142" = 5.8
  dimension "d143" = 5.8
  dimension "d144" = 5.8
  constraint vertical L0
  constraint coincident origin L0
  constraint horizontal L1
  constraint coincident origin L1
  constraint perpendicular L1 L2
  constraint perpendicular L1 L3
  constraint perpendicular L3 L4
  constraint perpendicular L3 L5
  constraint perpendicular L3 L6
  constraint perpendicular L2 L7
  constraint coincident L2 P12
  constraint coincident L6 P12
  constraint coincident L2 P11
  constraint coincident L7 P11
  constraint coincident L8 P2
  constraint coincident L9 P2
  constraint coincident L7 P10
  constraint coincident L3 P10
  constraint coincident L6 P13
  constraint coincident L3 P13
  constraint coincident L9 P13
  constraint coincident L9 P11
  constraint coincident L8 P10
  constraint coincident L8 P12
  constraint coincident L2 P15
  constraint coincident L5 P15
  constraint coincident L3 P14
  constraint coincident L5 P14
  constraint coincident L3 P17
  constraint coincident L4 P17
  constraint coincident L2 P16
  constraint coincident L4 P16
  constraint coincident P15 L10
  constraint coincident P17 L10
  constraint coincident P16 L11
  constraint coincident P14 L11
  constraint midpoint L10 P9
  constraint coincident P9 A0.centre
  constraint coincident P2 A1.centre
  constraint coincident P17 P7
  constraint coincident P14 P6
  constraint coincident P15 P5
  constraint coincident P16 P8
  constraint coincident P10 P3
  constraint coincident P11 P1
  constraint coincident P12 P0
  constraint coincident P13 P4
  constraint coincident L11 P9
  constraint horizontal L53
  constraint horizontal L59
  constraint horizontal L41
  constraint horizontal L47
  constraint horizontal L29
  constraint horizontal L35
  constraint horizontal L23
  constraint horizontal L17
  constraint horizontal L60
  constraint vertical L61
  constraint horizontal L62
  constraint vertical L63
  constraint horizontal L64
  constraint vertical L65
  constraint horizontal L66
  constraint vertical L67
  constraint horizontal L68
  constraint vertical L69
  constraint horizontal L70
  constraint vertical L71
  constraint horizontal L72
  constraint vertical L73
  constraint horizontal L74
  constraint vertical L75
  constraint horizontal L76
  constraint vertical L77
  constraint horizontal L78
  constraint vertical L79
  constraint horizontal L80
  constraint vertical L81
  constraint horizontal L82
  constraint vertical L83
  constraint horizontal L84
  constraint vertical L85
  constraint horizontal L86
  constraint vertical L87
  constraint horizontal L88
  constraint vertical L89
  constraint horizontal L90
  constraint vertical L91
  constraint coincident L23 L22.end
  constraint coincident L21.end L89
  constraint coincident L17 L16.end
  constraint coincident L15.end L85
  constraint coincident L27.end L77
  constraint coincident L33.end L81
  constraint coincident L35 L34.end
  constraint coincident L29 L28.end
  constraint coincident L53 L52.end
  constraint coincident L51.end L61
  constraint coincident L59 L58.end
  constraint coincident L57.end L65
  constraint coincident L41 L40.end
  constraint coincident L39.end L69
  constraint coincident L45.end L73
  constraint coincident L47 L46.end
  measures "d121" distance of L0 L2
  measures "d122" distance of L2 L3
  measures "d123" distance of L1 L4
  measures "d124" distance of L4 L5
  measures "d125" distance of L5 L6
  measures "d126" distance of L6 L7
  measures "d127" diameter of A1
  measures "d128" diameter of A0
  measures "d129" diameter of A6
  measures "d130" diameter of A7
  measures "d131" diameter of A8
  measures "d132" diameter of A9
  measures "d133" diameter of A3
  measures "d134" diameter of A4
  measures "d135" diameter of A2
  measures "d136" diameter of A5
  measures "d137" distance of L14 L17
  measures "d138" distance of L32 L35
  measures "d139" distance of L26 L29
  measures "d140" distance of L20 L23
  measures "d141" distance of L44 L47
  measures "d142" distance of L38 L41
  measures "d143" distance of L56 L59
  measures "d144" distance of L50 L53
extrude "Extrusion16" cut sketch "Skizze5" along normal blind 15 contours A2 L67 | A2 L67 | A3 L71 | A3 L71 | A4 L75 | A4 L75 | A5 L63 | A5 L63 | A6 L87 | A6 L87 | A7 L91 | A7 L91 | A8 L79 | A8 L79 | A9 L83 | A9 L83
extrude "Extrusion17" cut sketch "Skizze5" along normal blind 2 contours A0 | A1
move_face "Flächen versetzen4" offset -0.2 2 faces at (-20.0571, 217.0537, 6.3333) (-19.7629, 22.1017, 5.6667)
extrude "Extrusion18" cut sketch "Skizze5" along normal blind 5.7 contours A2 L54 L55 L56 L59 L67 | A2 L57 L58 L67 | L57 L64 L65 | L58 L65 L66 | A3 L36 L37 L38 L41 L71 | A3 L39 L40 L71 | L39 L68 L69 | L40 L69 L70 | A4 L42 L43 L44 L47 L75 | A4 L45 L46 L75 | L45 L72 L73 | L46 L73 L74 | A5 L48 L49 L50 L53 L63 | A5 L51 L52 L63 | L51 L60 L61 | L52 L61 L62 | A6 L12 L13 L14 L17 L87 | A6 L15 L16 L87 | L15 L84 L85 | L16 L85 L86 | A7 L18 L19 L20 L23 L91 | A7 L21 L22 L91 | L21 L88 L89 | L22 L89 L90 | A8 L24 L25 L26 L29 L79 | A8 L27 L28 L79 | L27 L76 L77 | L28 L77 L78 | A9 L30 L31 L32 L35 L83 | A9 L33 L34 L83 | L33 L80 L81 | L34 L81 L82
extrude "Extrusion19" add sketch "Skizze5" along normal blind 3 contours A2 L54 L55 L56 L59 L67 | A2 L57 L58 L67 | L57 L64 L65 | L58 L65 L66 | A3 L36 L37 L38 L41 L71 | A3 L39 L40 L71 | L39 L68 L69 | L40 L69 L70 | A4 L42 L43 L44 L47 L75 | A4 L45 L46 L75 | L45 L72 L73 | L46 L73 L74 | A5 L48 L49 L50 L53 L63 | A5 L51 L52 L63 | L51 L60 L61 | L52 L61 L62 | A6 L12 L13 L14 L17 L87 | A6 L15 L16 L87 | L15 L84 L85 | L16 L85 L86 | A7 L18 L19 L20 L23 L91 | A7 L21 L22 L91 | L21 L88 L89 | L22 L89 L90 | A8 L24 L25 L26 L29 L79 | A8 L27 L28 L79 | L27 L76 L77 | L28 L77 L78 | A9 L30 L31 L32 L35 L83 | A9 L33 L34 L83 | L33 L80 L81 | L34 L81 L82
extrude "Extrusion20" cut sketch "Skizze2" along normal blind 5 contours L66 L67 L68 L70 L71 A4 A11 A12
extrude "Extrusion21" add sketch "Skizze2" against normal blind 6 contours A7 | A8 | L74 L75 L76 L77 L78 L79 | L80 L81 L82 L83 L84 L85 | A14 | A16 | A18 | L95 L96 L97 L98 L99 L100 | L101 L102 L103 L104 L105 L106 | L107 L108 L109 L110 L111 L112
extrude "Extrusion22" add sketch "Skizze2" against normal blind 4 contours A5 | A6
extrude "Extrusion23" cut sketch "Skizze2" against normal blind 1.8 contours L74 L75 L76 L77 L78 L79 | L80 L81 L82 L83 L84 L85 | L95 L96 L97 L98 L99 L100 | L101 L102 L103 L104 L105 L106 | L107 L108 L109 L110 L111 L112
extrude "Extrusion24" cut sketch "Skizze2" along normal blind 4 contours A9 | A10 | A13 | A15 | A17
move_face "Flächen versetzen5" offset -0.2 1 faces at (-6.5763, 79.3333, 53.585)
equation "d162 = ( 2.5 * 2.54 ) * 1 mm"
equation "d165 = ( 2.5 * 2.54 ) * 1 mm"
named bodies: "side_right"
